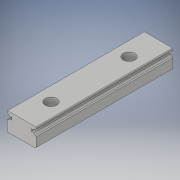
# Autodesk Inventor part: SSEBZ-MX16-70_r
Saved by Autodesk Inventor 2019 (Build 230136000, 136)
## iProperties
Created: 2022-12-29
Part Number: SSEBZ-MX16-70_r
Material: Generic
Catalog Web Link: www.cadenas.de
Description: SSEBZ, SSEBZ-MX, SSE2BZ, SSE2BZ-MX, SSEBLZ, SSEBLZ-MX, SSE2BLZ, SSE2BLZ-MX, SEBZ, SE2BZ, SEBLZ, SE2BLZ_rail-Miniature Linear Guides - Standard Blocks - Light Preload/Slight Clearance - Standard Grade - Selectable/Configurable
Vendor: MISUMI
Document SubType Name: Modeling
Designer: psAdmin
Manufacturer: MISUMI
Mass: 8.93148 g
Surface Area: 43.8495 cm^2
Volume: 8.93148 cm^3
Density: 1 g/cm^3
Appearance: PSOLRGB-175-175-175
Category: PARTsolutions
Company: MISUMI
Title: SSEBZ-MX16-70
Author: Cadenas PARTsolutions
Comments: Miniature Linear Guides - Standard Blocks - Light Preload/Slight Clearance - Standard Grade - Selectable/Configurable
PSOL_IDENT_0: {$CADENAS_DATA/23d-libs/misumi/metric/06_linear_guides/ssebz_series/sebz_rail.prj},303 {VTYP=3D},{NB=
PSOL_IDENT_1: SSEBZ-MX16-70_r},{LINA=SSEBZ-MX16-70},{NN=SSEBZ, SSEBZ-MX, SSE2BZ, SSE2BZ-MX, SSEBLZ, SSEBLZ-MX, SSE
PSOL_IDENT_2: 2BLZ, SSE2BLZ-MX, SEBZ, SE2BZ, SEBLZ, SE2BLZ_rail},{DATE=17.02.2022 00:39:33},{GEOMDATE=20.01.2022 0
PSOL_IDENT_3: 8:28:16},{VERSION=},{LINEID=300},{WBVAR=MAT,MX,NOB,LT,LS,ALT1,ALT2,ALT4},{WBNUMERIC=LS}  {NB=SSEBZ-M
PSOL_IDENT_4: X16-70_r},{LINA=SSEBZ-MX16-70},{KT=DUMMY},{PN=SSEBZ-MX16-70},{RT=B},{TS=Z},{TYPE=SSEBZ},{MAT=S},{MXA
PSOL_IDENT_5: LG='', 'w/o MX(Lubrication unit)', '-MX', 'with MX(Lubrication unit)'},{MX=-MX},{NOB=},{H=16},{LT=Se
PSOL_IDENT_6: lectable},{LTALG='Selectable','Selectable','Configurable','Configurable'},{LS=70},{W=32},{L1=42.4},{
PSOL_IDENT_7: B=25},{C=20},{S=M3x4},{L2=27.4},{K=12.0},{CBB=0.5},{W1=15},{W2=8.5},{H1=9.5},{CAA=0.5},{DD1DD2HH=3.5
PSOL_IDENT_8: x6x4.5},{F=40},{G=15.0},{DD2=6.000},{HH=4.500},{DD1=3.500},{ALT1=},{MC=M5},{MC1=5},{ALT2=},{ALT2L=10
PSOL_IDENT_9: .0},{ALT2N=5},{M=2},{LL=},{L0=70,110,150,190,230,270,310,350,390,430,470,510,550,590,630,670,710,750
PSOL_IDENT_10: ,790,830,870,910,950,990},{REC1=   '','w/o Rail Ends Cut alteration','-LLC','with LLC (Left End Cut)'
PSOL_IDENT_11: ,'-RLC','with RLC (Right End Cut)','-LLC-RLC','with Both End Cut'   },{MAT2='','Carbon Steel','S','S
PSOL_IDENT_12: tainless Steel'},{NL=0.000},{ALT4=},{ALT4ALG= '','Not applicable' },{CA1=0.3},{CA2=0.5},{VA1=2.5},{H
PSOL_IDENT_13: A1=2.5},{HA2=15.6300},{WA1=3.4477},{WA2=1.2},{RA1=3.50},{POIA1=0.2300},{NA1=1}
NB: SSEBZ-MX16-70_r
NN: SSEBZ, SSEBZ-MX, SSE2BZ, SSE2BZ-MX, SSEBLZ, SSEBLZ-MX, SSE2BLZ, SSE2BLZ-MX, SEBZ, SE2BZ, SEBLZ, SE2BLZ_rail
NT: Miniature Linear Guides - Standard Blocks - Light Preload/Slight Clearance - Standard Grade - Selectable/Configurable
NBSYN: $PN._r
LINA: SSEBZ-MX16-70
CATALOG: Misumi
PN: SSEBZ-MX16-70
MAT: Stainless Steel
MX: with MX(Lubrication unit)
NOB: 1
H: 16
LT: Selectable
LS: 70
W: 32
L1: 42.4
B: 25
C: 20
S: M3x4
L2: 27.4
K: 12
CBB: 0.5
W1: 15
W2: 8.5
H1: 9.5
CAA: 0.5
DD1DD2HH: 3.5x6x4.5
F: 40
G: 15
ALT1: w/o MC (Tapped Holes)
ALT2: w/o Rail Ends Cut alteration
ALT4: Not applicable
SUPPLIER: MISUMI
ARTICLENO: SSEBZ-MX16-70_r
BOMINFO: SSEBZ-MX16-70
CREATOR: CADENAS GmbH
Autodesk Inventor part; units mm, degrees
sketch "Sketch_12" plane through (0, 0, 0) normal (0, 0, 1) x (1, 0, 0)
  line L0 (-7.5, 9.2) -> (-7.5, 8.7239)
  line L1 (-7.5, 8.7239) -> (-6.94, 8.4006)
  arc A0 (-6.2177, 7.6) -> (-6.94, 8.4006) centre (-7.815, 6.885) ccw
  line L2 (-6.2177, 7.6) -> (-5, 7.6)
  line L3 (-5, 7.6) -> (-5, 6.4)
  line L4 (-5, 6.4) -> (-6.2177, 6.4)
  arc A1 (-6.94, 5.5994) -> (-6.2177, 6.4) centre (-7.815, 7.115) ccw
  line L5 (-6.94, 5.5994) -> (-7.5, 5.2762)
  line L6 (-7.5, 5.2762) -> (-7.5, 0.5)
  line L7 (-7.5, 0.5) -> (-7, 0)
  line L8 (-7, 0) -> (7, 0)
  line L9 (7, 0) -> (7.5, 0.5)
  line L10 (7.5, 0.5) -> (7.5, 5.2762)
  line L11 (7.5, 5.2762) -> (6.94, 5.5994)
  arc A2 (6.2177, 6.4) -> (6.94, 5.5994) centre (7.815, 7.115) ccw
  line L12 (6.2177, 6.4) -> (5, 6.4)
  line L13 (5, 6.4) -> (5, 7.6)
  line L14 (5, 7.6) -> (6.2177, 7.6)
  arc A3 (6.94, 8.4006) -> (6.2177, 7.6) centre (7.815, 6.885) ccw
  line L15 (6.94, 8.4006) -> (7.5, 8.7239)
  line L16 (7.5, 8.7239) -> (7.5, 9.2)
  line L17 (7.5, 9.2) -> (7.2, 9.5)
  line L18 (7.2, 9.5) -> (-7.2, 9.5)
  line L19 (-7.2, 9.5) -> (-7.5, 9.2)
  constraints: 40 end point, 8 point on circle, 4 centre point
extrude "Extrusion1" add sketch "Sketch_12" along normal mid plane 70
sketch "Sketch2" plane through (-7.2, 9.5, 35) normal (0, 1, 0) x (1, 0, 0)
  point P0 (7.2, 55)
hole "Hole1" at (0, 9.5, -20) direction (0, -1, 0) diameter 3.5 depth 9.5 counterbore diameter 6 counterbore depth 4.5
pattern_linear "Rectangular Pattern1" count 2 spacing 40 along (0, 0, 1) of "Hole1"
ref_plane "to_block_XY" through (0, 9.5, 0) normal (0, 0, 1) x (1, 0, 0)
ref_plane "to_block_YZ" through (0, 9.5, 0) normal (1, 0, 0) x (0, 1, 0)
ref_plane "to_block_ZX" through (0, 9.5, 0) normal (0, 1, 0) x (0, 0, 1)
body "Solid1"
